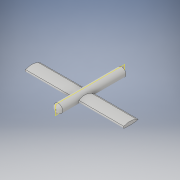
# Autodesk Inventor part: airfoil
Saved by Autodesk Inventor 2017 (Build 210142000, 142)
## iProperties
Created: 2019-04-05
Part Number: airfoil
Material: Generic
Document SubType Name: Modeling
Designer: qthuynh
Density: 1 g/cm^3
Appearance: Default
Author: qthuynh
Autodesk Inventor part; units mm, degrees
ref_plane "XZ Plane" through (0, 0, 0) normal (0, 1, 0) x (-1, 0, 0)
ref_plane "XY Plane" through (0, 0, 0) normal (0, 0, 1) x (1, 0, 0)
sketch "Sketch1" plane through (0, 0, 0) normal (0, 0, 1) x (1, 0, 0)
  circle A0 centre (0, 0) radius 10.4497
  constraints: 1 centre point, 1 coincident
extrude "Extrusion1" add sketch "Sketch1" along normal blind 152.4
ref_plane "Work Plane1" through (0, 0, 0) normal (1, 0, 0) x (0, 1, 0)
sketch "Sketch2" plane through (0, 0, 0) normal (1, 0, 0) x (0, 1, 0)
  arc A0 (1.8381, 82.7135) -> (2.0423, 113.1439) centre (-31.7521, 98.1548) ccw
  arc A1 (-2.6484, 112.1932) -> (-2.2475, 82.7136) centre (118.2266, 99.0943) ccw
  arc A2 (2.0423, 113.1439) -> (-2.6484, 112.1932) centre (-0.1518, 111.9227) ccw
  line L0 (1.8381, 82.7135) -> (-0.6507, 78.169)
  line L1 (-0.6507, 78.169) -> (-2.2475, 82.7136)
  point P0 (0, 0)
  constraints: 6 point on circle, 4 end point, 3 centre point, 1 tangent
extrude "Extrusion2" add sketch "Sketch2" along normal mid plane 236.5375 draft -0.1
sketch "Sketch3" plane through (0, 0, 152.4) normal (0, 0, 1) x (1, 0, 0)
  circle A0 centre (0, 0) radius 10.4497
  constraints: 1 centre point, 1 coincident
extrude "Extrusion3" add sketch "Sketch3" along normal mid plane 12.7 draft -0.1
fillet "Fillet1" radius 10.16 1 edges at (-10.4386, 0, 158.75)
body "Solid1"
